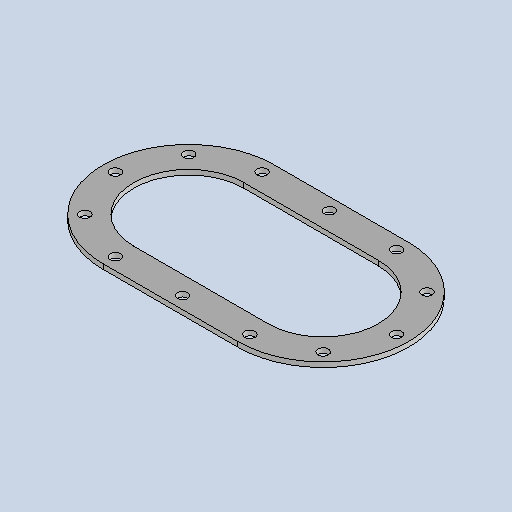
# Autodesk Inventor part: PNS-731 charging flange
Saved by Autodesk Inventor 2025.1 (Build 291241020, 241B)
## iProperties
Created: 2025-02-13
Part Number: PNS-731 charging flange
Material: Steel
Document SubType Name: Sheet Metal
Designer: pokla
Density: 7.85 g/cm^3
Sheet Metal Rule: AISI304 4mm Die 32
Sheet Metal Width: 0,000 mm
Sheet Metal Length: 0,000 mm
Sheet Metal Area: 0,000 mm^2
Appearance: Default
Author: pokla
Autodesk Inventor part; units mm, degrees
note: some values were not read from the file. Chosen so that the rebuilt part matches the saved one: pattern direction of "Circular Pattern1".
ref_plane "YZ Plane" through (0, 0, 0) normal (1, 0, 0) x (0, 1, 0)
ref_plane "XZ Plane" through (0, 0, 0) normal (0, 1, 0) x (-1, 0, 0)
ref_plane "XY Plane" through (0, 0, 0) normal (0, 0, 1) x (1, 0, 0)
sketch "Sketch2" plane through (0, 0, 0) normal (0, 0, 1) x (1, 0, 0)
  line L0 (-110, 0) -> (110, 0) construction
  line L1 (-110, -90) -> (110, -90)
  line L2 (110, 90) -> (-110, 90)
  arc A0 (-110, 90) -> (-110, -90) centre (-110, 0) ccw
  arc A1 (110, -90) -> (110, 90) centre (110, 0) ccw
  line L3 (-200, 0) -> (200, 0) construction
  line L4 (-110, 140) -> (110, 140)
  arc A2 (110, -140) -> (110, 140) centre (110, 0) ccw
  line L5 (110, -140) -> (-110, -140)
  arc A3 (-110, 140) -> (-110, -140) centre (-110, 0) ccw
  point P0 (0, 0)
  dimension "Charging_hatch_width" = 400
  dimension "d11" = 400
  dimension "d12" = 180
  dimension "d13" = 50
  measures "d11" distance of L3.start L3.end
  measures "d12" distance between parallel lines of L1 L2
  measures "d13" distance between parallel lines of L2 L4
extrude "Plate2" add sketch "Sketch2" along normal blind 8
sketch "Sketch3" plane through (0, 0, 8) normal (0, 0, 1) x (1, 0, 0)
  arc A0 (-110, 140) -> (-110, -140) centre (-110, 0) ccw construction
  line L0 (-110, 140) -> (110, 140) construction
  arc A1 (110, -140) -> (110, 140) centre (110, 0) ccw construction
  line L1 (110, -140) -> (-110, -140) projected
  circle A2 centre (-230, 0) radius 8.5
  arc A3 (-110, 120) -> (-110, -120) centre (-110, 0) ccw construction
  line L2 (-110, 120) -> (110, 120) construction
  arc A4 (110, -120) -> (110, 120) centre (110, 0) ccw construction
  line L3 (110, -120) -> (-110, -120) construction
  point P0 (0, 0)
  dimension "Charging_hatch_width" = 400
  dimension "d15" = 17
  dimension "d16" = 20
  constraints: 5 point on circle, 4 end point, 3 centre point, 1 horizontal alignment, 3 other
  measures "d15" diameter of A2
  measures "d16" radial gap between concentric circles of A0 A3
extrude "Cut1" cut sketch "Sketch3" against normal blind 8
pattern_circular "Circular Pattern1" count 5 over 180 about axis through (-110, 0, 0) along (0, 0, 1) of "Cut1" both ways yes
mirror "Mirror1" about plane through (0, 0, 0) normal (1, 0, 0) of "Cut1", "Circular Pattern1"
sketch "Sketch4" plane through (0, 0, 8) normal (0, 0, 1) x (1, 0, 0)
  circle A0 centre (-110, 120) radius 8.5 construction
  circle A1 centre (110, 120) radius 8.5 construction
  circle A2 centre (-110, -120) radius 8.5 construction
  circle A3 centre (110, -120) radius 8.5 construction
  circle A4 centre (0, -120) radius 8.5
  circle A5 centre (0, 120) radius 8.5
  point P0 (0, 0)
  dimension "Charging_hatch_width" = 400
  dimension "d22" = 0
  constraints: 2 centre point, 2 equal radius, 2 horizontal alignment, 1 vertical alignment
  measures "d22" horizontal distance of point (0, 0) A5.centre
extrude "Cut2" cut sketch "Sketch4" against normal blind 8
equation "\"d11\" = Charging_hatch_width"
equation "\"d12\" = Charging_hatch_hight"
equation "\"d17\" = Thickness"
equation "\"d23\" = Thickness"
equation "\"d14\" = Thickness"
equation "\"BendReliefWidth\" = Thickness"
equation "\"BendReliefDepth\" = 0.5 * Thickness"
equation "\"CornerReliefSize\" = 4 * Thickness"
equation "\"MinimumRemnant\" = 2 * Thickness"
equation "\"TransitionRadius\" = BendRadius"
equation "\"JacobiRadiusSize\" = BendRadius"
equation "\"GapSize\" = Thickness"
equation "\"Charging_hatch_hight\" = 180"
equation "\"Thickness\" = 8"
equation "\"BendRadius\" = 6"
body "Solid3"
